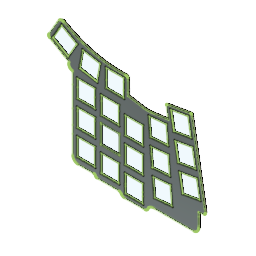
Klein-switchplate-MX-v2 (Autodesk Fusion 360 design; units mm, degrees)
Autodesk Fusion 360 part; units mm, degrees
note: some values were not read from the file. Set by a fixed rule: which sketch regions a step uses.
sketch "Sketch1" plane through (0, 0, 0) normal (0, 1, 0) x (1, 0, 0)
  line L0 (58.9921, 32.8367) -> (59.0035, 32.7548)
  line L1 (59.0035, 32.7548) -> (59.0201, 32.6338)
  line L2 (59.0201, 32.6338) -> (59.0381, 32.4299)
  line L3 (59.0381, 32.4299) -> (59.0461, 32.226)
  line L4 (59.0461, 32.226) -> (59.0441, 32.0221)
  line L5 (59.0441, 32.0221) -> (59.0321, 31.8171)
  line L6 (59.0321, 31.8171) -> (59.0321, 30.7985)
  line L7 (59.0321, 30.7985) -> (59.0321, 24.5661)
  line L8 (59.0321, 24.5661) -> (59.0321, 21.4739)
  line L9 (59.0321, 21.4739) -> (59.0321, 21.4713)
  line L10 (59.0321, 21.4713) -> (63.4304, 20.5717)
  line L11 (63.4304, 20.5717) -> (63.484, 20.5607)
  line L12 (63.484, 20.5607) -> (63.5246, 20.5516)
  line L13 (63.5246, 20.5516) -> (63.6297, 20.5186)
  line L14 (63.6297, 20.5186) -> (63.6613, 20.5077)
  line L15 (63.6613, 20.5077) -> (63.7388, 20.4717)
  line L16 (63.7388, 20.4717) -> (63.7582, 20.4627)
  line L17 (63.7582, 20.4627) -> (63.8502, 20.4087)
  line L18 (63.8502, 20.4087) -> (63.9371, 20.3458)
  line L19 (63.9371, 20.3458) -> (63.9921, 20.297)
  line L20 (63.9921, 20.297) -> (64.0199, 20.272)
  line L21 (64.0199, 20.272) -> (64.0577, 20.2321)
  line L22 (64.0577, 20.2321) -> (64.088, 20.1975)
  line L23 (64.088, 20.1975) -> (64.1341, 20.1404)
  line L24 (64.1341, 20.1404) -> (64.1528, 20.1129)
  line L25 (64.1528, 20.1129) -> (64.2105, 20.0188)
  line L26 (64.2105, 20.0188) -> (64.2396, 19.9588)
  line L27 (64.2396, 19.9588) -> (64.263, 19.9093)
  line L28 (64.263, 19.9093) -> (64.2884, 19.8399)
  line L29 (64.2884, 19.8399) -> (64.3024, 19.7918)
  line L30 (64.3024, 19.7918) -> (64.3258, 19.6942)
  line L31 (64.3258, 19.6942) -> (64.3308, 19.6611)
  line L32 (64.3308, 19.6611) -> (64.3404, 19.5786)
  line L33 (64.3404, 19.5786) -> (64.3423, 19.5287)
  line L34 (64.3423, 19.5287) -> (64.3409, 19.4276)
  line L35 (64.3409, 19.4276) -> (64.3369, 19.3861)
  line L36 (64.3369, 19.3861) -> (64.33, 19.3222)
  line L37 (64.33, 19.3222) -> (63.8116, 16.3774)
  line L38 (63.8116, 16.3774) -> (60.9284, 0)
  line L39 (60.9284, 0) -> (58.0453, -16.3774)
  line L40 (58.0453, -16.3774) -> (57.1727, -21.3338)
  line L41 (57.1727, -21.3338) -> (55.1621, -32.7548)
  line L42 (55.1621, -32.7548) -> (53.7066, -41.0228)
  line L43 (53.7066, -41.0228) -> (53.3844, -42.8527)
  line L44 (53.3844, -42.8527) -> (53.3634, -42.9266)
  line L45 (53.3634, -42.9266) -> (53.3314, -43.0046)
  line L46 (53.3314, -43.0046) -> (53.3208, -43.0234)
  line L47 (53.3208, -43.0234) -> (53.2878, -43.0776)
  line L48 (53.2878, -43.0776) -> (53.275, -43.0951)
  line L49 (53.275, -43.0951) -> (53.2462, -43.1322)
  line L50 (53.2462, -43.1322) -> (53.228, -43.1516)
  line L51 (53.228, -43.1516) -> (53.1702, -43.2062)
  line L52 (53.1702, -43.2062) -> (53.1662, -43.21)
  line L53 (53.1662, -43.21) -> (53.1318, -43.2341)
  line L54 (53.1318, -43.2341) -> (53.0976, -43.2589)
  line L55 (53.0976, -43.2589) -> (53.0931, -43.2622)
  line L56 (53.0931, -43.2622) -> (53.0223, -43.2972)
  line L57 (53.0223, -43.2972) -> (53.0051, -43.306)
  line L58 (53.0051, -43.306) -> (52.978, -43.3154)
  line L59 (52.978, -43.3154) -> (52.9326, -43.3305)
  line L60 (52.9326, -43.3305) -> (52.8646, -43.3455)
  line L61 (52.8646, -43.3455) -> (52.8384, -43.3477)
  line L62 (52.8384, -43.3477) -> (52.749, -43.3525)
  line L63 (52.749, -43.3525) -> (52.7347, -43.3525)
  line L64 (52.7347, -43.3525) -> (49.1321, -42.728)
  line L65 (49.1321, -42.728) -> (36.5731, -40.551)
  line L66 (36.5731, -40.551) -> (33.9933, -40.1038)
  line L67 (33.9933, -40.1038) -> (33.9483, -40.0888)
  line L68 (33.9483, -40.0888) -> (33.8709, -40.0528)
  line L69 (33.8709, -40.0528) -> (33.8623, -40.0488)
  line L70 (33.8623, -40.0488) -> (33.8273, -40.0261)
  line L71 (33.8273, -40.0261) -> (33.7881, -39.9931)
  line L72 (33.7881, -39.9931) -> (33.759, -39.9722)
  line L73 (33.759, -39.9722) -> (33.7375, -39.9488)
  line L74 (33.7375, -39.9488) -> (33.7004, -39.9069)
  line L75 (33.7004, -39.9069) -> (33.6654, -39.8569)
  line L76 (33.6654, -39.8569) -> (33.6284, -39.7849)
  line L77 (33.6284, -39.7849) -> (33.6014, -39.7089)
  line L78 (33.6014, -39.7089) -> (33.589, -39.6354)
  line L79 (33.589, -39.6354) -> (33.5834, -39.5998)
  line L80 (33.5834, -39.5998) -> (33.5903, -39.4981)
  line L81 (33.5903, -39.4981) -> (33.5906, -39.4728)
  line L82 (33.5906, -39.4728) -> (33.5931, -39.4558)
  line L83 (33.5931, -39.4558) -> (33.5934, -39.454)
  line L84 (33.5934, -39.454) -> (34.7453, -32.7548)
  line L85 (34.7453, -32.7548) -> (35.1918, -30.1578)
  line L86 (35.1918, -30.1578) -> (32.7548, -29.8255)
  line L87 (32.7548, -29.8255) -> (23.4475, -28.5565)
  line L88 (23.4475, -28.5565) -> (22.1161, -28.3575)
  line L89 (22.1161, -28.3575) -> (21.6487, -28.3112)
  line L90 (21.6487, -28.3112) -> (20.7756, -28.2246)
  line L91 (20.7756, -28.2246) -> (19.4311, -28.1586)
  line L92 (19.4311, -28.1586) -> (18.0847, -28.1576)
  line L93 (18.0847, -28.1576) -> (16.7402, -28.2246)
  line L94 (16.7402, -28.2246) -> (15.4008, -28.3565)
  line L95 (15.4008, -28.3565) -> (2.9558, -30.4057)
  line L96 (2.9558, -30.4057) -> (2.9358, -32.7548)
  line L97 (2.9358, -32.7548) -> (2.866, -40.9434)
  line L98 (2.866, -40.9434) -> (2.8498, -42.8427)
  line L99 (2.8498, -42.8427) -> (2.8019, -42.9236)
  line L100 (2.8019, -42.9236) -> (2.7566, -42.9906)
  line L101 (2.7566, -42.9906) -> (2.7229, -43.0406)
  line L102 (2.7229, -43.0406) -> (2.6359, -43.1526)
  line L103 (2.6359, -43.1526) -> (2.5926, -43.2007)
  line L104 (2.5926, -43.2007) -> (2.5523, -43.2438)
  line L105 (2.5523, -43.2438) -> (2.507, -43.2905)
  line L106 (2.507, -43.2905) -> (2.402, -43.3845)
  line L107 (2.402, -43.3845) -> (2.2901, -43.4714)
  line L108 (2.2901, -43.4714) -> (2.1721, -43.5494)
  line L109 (2.1721, -43.5494) -> (2.0482, -43.6184)
  line L110 (2.0482, -43.6184) -> (2.0472, -43.6188)
  line L111 (2.0472, -43.6188) -> (2.0216, -43.6312)
  line L112 (2.0216, -43.6312) -> (1.9034, -43.6848)
  line L113 (1.9034, -43.6848) -> (1.8488, -43.7063)
  line L114 (1.8488, -43.7063) -> (1.7883, -43.7283)
  line L115 (1.7883, -43.7283) -> (1.6523, -43.7683)
  line L116 (1.6523, -43.7683) -> (1.5144, -43.7993)
  line L117 (1.5144, -43.7993) -> (1.3734, -43.8183)
  line L118 (1.3734, -43.8183) -> (1.2325, -43.8283)
  line L119 (1.2325, -43.8283) -> (1.0916, -43.8263)
  line L120 (1.0916, -43.8263) -> (0.9506, -43.8153)
  line L121 (0.9506, -43.8153) -> (0.8567, -43.8013)
  line L122 (0.8567, -43.8013) -> (0.7395, -43.7988)
  line L123 (0.7395, -43.7988) -> (0, -43.7832)
  line L124 (0, -43.7832) -> (-3.3556, -43.7123)
  line L125 (-3.3556, -43.7123) -> (-7.5679, -43.8223)
  line L126 (-7.5679, -43.8223) -> (-11.7702, -44.1302)
  line L127 (-11.7702, -44.1302) -> (-15.9535, -44.637)
  line L128 (-15.9535, -44.637) -> (-20.1079, -45.3407)
  line L129 (-20.1079, -45.3407) -> (-24.2242, -46.2403)
  line L130 (-24.2242, -46.2403) -> (-28.2936, -47.3329)
  line L131 (-28.2936, -47.3329) -> (-32.3069, -48.6163)
  line L132 (-32.3069, -48.6163) -> (-32.7548, -48.7832)
  line L133 (-32.7548, -48.7832) -> (-33.691, -49.1321)
  line L134 (-33.691, -49.1321) -> (-36.2553, -50.0877)
  line L135 (-36.2553, -50.0877) -> (-40.1298, -51.7441)
  line L136 (-40.1298, -51.7441) -> (-43.9222, -53.5823)
  line L137 (-43.9222, -53.5823) -> (-47.6227, -55.5975)
  line L138 (-47.6227, -55.5975) -> (-47.7467, -55.6825)
  line L139 (-47.7467, -55.6825) -> (-47.9406, -55.7984)
  line L140 (-47.9406, -55.7984) -> (-48.1415, -55.9014)
  line L141 (-48.1415, -55.9014) -> (-48.2893, -55.9605)
  line L142 (-48.2893, -55.9605) -> (-48.334, -55.9784)
  line L143 (-48.334, -55.9784) -> (-48.3774, -55.9968)
  line L144 (-48.3774, -55.9968) -> (-48.3976, -56.0038)
  line L145 (-48.3976, -56.0038) -> (-48.4664, -56.0277)
  line L146 (-48.4664, -56.0277) -> (-48.5654, -56.0593)
  line L147 (-48.5654, -56.0593) -> (-48.7843, -56.1133)
  line L148 (-48.7843, -56.1133) -> (-49.0072, -56.1533)
  line L149 (-49.0072, -56.1533) -> (-49.1321, -56.1641)
  line L150 (-49.1321, -56.1641) -> (-49.3071, -56.1793)
  line L151 (-49.3071, -56.1793) -> (-49.533, -56.1783)
  line L152 (-49.533, -56.1783) -> (-49.7579, -56.1633)
  line L153 (-49.7579, -56.1633) -> (-49.9818, -56.1293)
  line L154 (-49.9818, -56.1293) -> (-50.2027, -56.0813)
  line L155 (-50.2027, -56.0813) -> (-50.3476, -56.0393)
  line L156 (-50.3476, -56.0393) -> (-50.5596, -55.9624)
  line L157 (-50.5596, -55.9624) -> (-50.7665, -55.8714)
  line L158 (-50.7665, -55.8714) -> (-50.8083, -55.8499)
  line L159 (-50.8083, -55.8499) -> (-50.9898, -55.7502)
  line L160 (-50.9898, -55.7502) -> (-51.0304, -55.7265)
  line L161 (-51.0304, -55.7265) -> (-51.2183, -55.6005)
  line L162 (-51.2183, -55.6005) -> (-51.3972, -55.4626)
  line L163 (-51.3972, -55.4626) -> (-51.6181, -55.2577)
  line L164 (-51.6181, -55.2577) -> (-51.7201, -55.1467)
  line L165 (-51.7201, -55.1467) -> (-52.8694, -53.2265)
  line L166 (-52.8694, -53.2265) -> (-53.2265, -52.6299)
  line L167 (-53.2265, -52.6299) -> (-55.32, -49.1321)
  line L168 (-55.32, -49.1321) -> (-59.6169, -41.953)
  line L169 (-59.6169, -41.953) -> (-59.6669, -41.8851)
  line L170 (-59.6669, -41.8851) -> (-59.7348, -41.7801)
  line L171 (-59.7348, -41.7801) -> (-59.8138, -41.6322)
  line L172 (-59.8138, -41.6322) -> (-59.8638, -41.5162)
  line L173 (-59.8638, -41.5162) -> (-59.8725, -41.4915)
  line L174 (-59.8725, -41.4915) -> (-59.9152, -41.3541)
  line L175 (-59.9152, -41.3541) -> (-59.9258, -41.3163)
  line L176 (-59.9258, -41.3163) -> (-59.9518, -41.1933)
  line L177 (-59.9518, -41.1933) -> (-59.9678, -41.0694)
  line L178 (-59.9678, -41.0694) -> (-59.9758, -40.9434)
  line L179 (-59.9758, -40.9434) -> (-59.9728, -40.8185)
  line L180 (-59.9728, -40.8185) -> (-59.9696, -40.7791)
  line L181 (-59.9696, -40.7791) -> (-59.9579, -40.6644)
  line L182 (-59.9579, -40.6644) -> (-59.9539, -40.6388)
  line L183 (-59.9539, -40.6388) -> (-59.9312, -40.5261)
  line L184 (-59.9312, -40.5261) -> (-59.9228, -40.4876)
  line L185 (-59.9228, -40.4876) -> (-59.8868, -40.3667)
  line L186 (-59.8868, -40.3667) -> (-59.8675, -40.3124)
  line L187 (-59.8675, -40.3124) -> (-59.8485, -40.2637)
  line L188 (-59.8485, -40.2637) -> (-59.8134, -40.1846)
  line L189 (-59.8134, -40.1846) -> (-59.7959, -40.1496)
  line L190 (-59.7959, -40.1496) -> (-59.7561, -40.0734)
  line L191 (-59.7561, -40.0734) -> (-59.7361, -40.0393)
  line L192 (-59.7361, -40.0393) -> (-59.6564, -39.9197)
  line L193 (-59.6564, -39.9197) -> (-59.6339, -39.8879)
  line L194 (-59.6339, -39.8879) -> (-59.5549, -39.7899)
  line L195 (-59.5549, -39.7899) -> (-59.468, -39.6989)
  line L196 (-59.468, -39.6989) -> (-59.376, -39.614)
  line L197 (-59.376, -39.614) -> (-59.3451, -39.5896)
  line L198 (-59.3451, -39.5896) -> (-59.2537, -39.5195)
  line L199 (-59.2537, -39.5195) -> (-59.2212, -39.4977)
  line L200 (-59.2212, -39.4977) -> (-59.1229, -39.4372)
  line L201 (-59.1229, -39.4372) -> (-59.1001, -39.4241)
  line L202 (-59.1001, -39.4241) -> (-57.3208, -38.4036)
  line L203 (-57.3208, -38.4036) -> (-49.1321, -33.7073)
  line L204 (-49.1321, -33.7073) -> (-47.4712, -32.7548)
  line L205 (-47.4712, -32.7548) -> (-43.5914, -30.5297)
  line L206 (-43.5914, -30.5297) -> (-43.6993, -30.3187)
  line L207 (-43.6993, -30.3187) -> (-43.729, -30.2506)
  line L208 (-43.729, -30.2506) -> (-43.8128, -30.0493)
  line L209 (-43.8128, -30.0493) -> (-43.8366, -29.9787)
  line L210 (-43.8366, -29.9787) -> (-43.8861, -29.8227)
  line L211 (-43.8861, -29.8227) -> (-43.9051, -29.7508)
  line L212 (-43.9051, -29.7508) -> (-43.9312, -29.645)
  line L213 (-43.9312, -29.645) -> (-43.9732, -29.4111)
  line L214 (-43.9732, -29.4111) -> (-43.9813, -29.3374)
  line L215 (-43.9813, -29.3374) -> (-44.002, -29.1209)
  line L216 (-44.002, -29.1209) -> (-44.0041, -29.0712)
  line L217 (-44.0041, -29.0712) -> (-44.0028, -28.8534)
  line L218 (-44.0028, -28.8534) -> (-44.0012, -28.7794)
  line L219 (-44.0012, -28.7794) -> (-43.9943, -28.7053)
  line L220 (-43.9943, -28.7053) -> (-43.9895, -28.6604)
  line L221 (-43.9895, -28.6604) -> (-43.971, -28.4882)
  line L222 (-43.971, -28.4882) -> (-43.9635, -28.4391)
  line L223 (-43.9635, -28.4391) -> (-43.9188, -28.2261)
  line L224 (-43.9188, -28.2261) -> (-43.9022, -28.1536)
  line L225 (-43.9022, -28.1536) -> (-43.8555, -27.9969)
  line L226 (-43.8555, -27.9969) -> (-43.8287, -27.9118)
  line L227 (-43.8287, -27.9118) -> (-43.8258, -27.9026)
  line L228 (-43.8258, -27.9026) -> (-43.7977, -27.8339)
  line L229 (-43.7977, -27.8339) -> (-43.7173, -27.6318)
  line L230 (-43.7173, -27.6318) -> (-43.6163, -27.438)
  line L231 (-43.6163, -27.438) -> (-43.5823, -27.3718)
  line L232 (-43.5823, -27.3718) -> (-43.5793, -27.367)
  line L233 (-43.5793, -27.367) -> (-43.5301, -27.2875)
  line L234 (-43.5301, -27.2875) -> (-43.4105, -27.1054)
  line L235 (-43.4105, -27.1054) -> (-43.3343, -27.0079)
  line L236 (-43.3343, -27.0079) -> (-43.2683, -26.9213)
  line L237 (-43.2683, -26.9213) -> (-43.2529, -26.9039)
  line L238 (-43.2529, -26.9039) -> (-43.1604, -26.799)
  line L239 (-43.1604, -26.799) -> (-43.1086, -26.7459)
  line L240 (-43.1086, -26.7459) -> (-43.0247, -26.6625)
  line L241 (-43.0247, -26.6625) -> (-42.9924, -26.6304)
  line L242 (-42.9924, -26.6304) -> (-42.9726, -26.6132)
  line L243 (-42.9726, -26.6132) -> (-42.91, -26.5589)
  line L244 (-42.91, -26.5589) -> (-42.7801, -26.46)
  line L245 (-42.7801, -26.46) -> (-42.6657, -26.3653)
  line L246 (-42.6657, -26.3653) -> (-42.529, -26.2753)
  line L247 (-42.529, -26.2753) -> (-42.511, -26.2639)
  line L248 (-42.511, -26.2639) -> (-42.4453, -26.2222)
  line L249 (-42.4453, -26.2222) -> (-42.3511, -26.1679)
  line L250 (-42.3511, -26.1679) -> (-42.1539, -26.0751)
  line L251 (-42.1539, -26.0751) -> (-42.0883, -26.0405)
  line L252 (-42.0883, -26.0405) -> (-42.043, -26.0205)
  line L253 (-42.043, -26.0205) -> (-41.8201, -25.9385)
  line L254 (-41.8201, -25.9385) -> (-41.6119, -25.8776)
  line L255 (-41.6119, -25.8776) -> (-41.5912, -25.8715)
  line L256 (-41.5912, -25.8715) -> (-41.3775, -25.8303)
  line L257 (-41.3775, -25.8303) -> (-41.3047, -25.8156)
  line L258 (-41.3047, -25.8156) -> (-41.2063, -25.8041)
  line L259 (-41.2063, -25.8041) -> (-41.0434, -25.7876)
  line L260 (-41.0434, -25.7876) -> (-40.9434, -25.7842)
  line L261 (-40.9434, -25.7842) -> (-40.8065, -25.7796)
  line L262 (-40.8065, -25.7796) -> (-40.8065, -24.5661)
  line L263 (-40.8065, -24.5661) -> (-40.8068, -16.3774)
  line L264 (-40.8068, -16.3774) -> (-40.8074, 0)
  line L265 (-40.8074, 0) -> (-40.8078, 11.4254)
  line L266 (-40.8078, 11.4254) -> (-40.808, 17.5229)
  line L267 (-40.808, 17.5229) -> (-40.8085, 31.5173)
  line L268 (-40.8085, 31.5173) -> (-40.8085, 32.167)
  line L269 (-40.8085, 32.167) -> (-40.8055, 32.3709)
  line L270 (-40.8055, 32.3709) -> (-40.7925, 32.5738)
  line L271 (-40.7925, 32.5738) -> (-40.772, 32.7548)
  line L272 (-40.772, 32.7548) -> (-40.7695, 32.7767)
  line L273 (-40.7695, 32.7767) -> (-40.7355, 32.9777)
  line L274 (-40.7355, 32.9777) -> (-40.6925, 33.1766)
  line L275 (-40.6925, 33.1766) -> (-40.6406, 33.3735)
  line L276 (-40.6406, 33.3735) -> (-40.5776, 33.5674)
  line L277 (-40.5776, 33.5674) -> (-40.5056, 33.7574)
  line L278 (-40.5056, 33.7574) -> (-40.4237, 33.9443)
  line L279 (-40.4237, 33.9443) -> (-40.3337, 34.1262)
  line L280 (-40.3337, 34.1262) -> (-40.2337, 34.3041)
  line L281 (-40.2337, 34.3041) -> (-40.1258, 34.4771)
  line L282 (-40.1258, 34.4771) -> (-40.0088, 34.644)
  line L283 (-40.0088, 34.644) -> (-39.8872, 34.8019)
  line L284 (-39.8872, 34.8019) -> (-39.8849, 34.8049)
  line L285 (-39.8849, 34.8049) -> (-39.7519, 34.9599)
  line L286 (-39.7519, 34.9599) -> (-39.612, 35.1068)
  line L287 (-39.612, 35.1068) -> (-39.465, 35.2477)
  line L288 (-39.465, 35.2477) -> (-39.3101, 35.3807)
  line L289 (-39.3101, 35.3807) -> (-39.1502, 35.5066)
  line L290 (-39.1502, 35.5066) -> (-38.9832, 35.6236)
  line L291 (-38.9832, 35.6236) -> (-38.8963, 35.6787)
  line L292 (-38.8963, 35.6787) -> (-38.8113, 35.7326)
  line L293 (-38.8113, 35.7326) -> (-38.6344, 35.8325)
  line L294 (-38.6344, 35.8325) -> (-38.4525, 35.9245)
  line L295 (-38.4525, 35.9245) -> (-38.2655, 36.0064)
  line L296 (-38.2655, 36.0064) -> (-38.0756, 36.0794)
  line L297 (-38.0756, 36.0794) -> (-37.8827, 36.1424)
  line L298 (-37.8827, 36.1424) -> (-37.6858, 36.1964)
  line L299 (-37.6858, 36.1964) -> (-37.4868, 36.2403)
  line L300 (-37.4868, 36.2403) -> (-37.2859, 36.2743)
  line L301 (-37.2859, 36.2743) -> (-37.084, 36.2983)
  line L302 (-37.084, 36.2983) -> (-36.8811, 36.3123)
  line L303 (-36.8811, 36.3123) -> (-36.8491, 36.3128)
  line L304 (-36.8491, 36.3128) -> (-36.6772, 36.3153)
  line L305 (-36.6772, 36.3153) -> (-32.7548, 36.3153)
  line L306 (-32.7548, 36.3153) -> (-24.5661, 36.3153)
  line L307 (-24.5661, 36.3153) -> (-24.2322, 36.3153)
  line L308 (-24.2322, 36.3153) -> (-24.1649, 36.3126)
  line L309 (-24.1649, 36.3126) -> (-24.1239, 36.3113)
  line L310 (-24.1239, 36.3113) -> (-24.0559, 36.3134)
  line L311 (-24.0559, 36.3134) -> (-24.039, 36.3153)
  line L312 (-24.039, 36.3153) -> (-23.9744, 36.3228)
  line L313 (-23.9744, 36.3228) -> (-23.8404, 36.3413)
  line L314 (-23.8404, 36.3413) -> (-23.8104, 36.3491)
  line L315 (-23.8104, 36.3491) -> (-23.6805, 36.3883)
  line L316 (-23.6805, 36.3883) -> (-23.6561, 36.3967)
  line L317 (-23.6561, 36.3967) -> (-23.6514, 36.3983)
  line L318 (-23.6514, 36.3983) -> (-23.5905, 36.4233)
  line L319 (-23.5905, 36.4233) -> (-23.4702, 36.4865)
  line L320 (-23.4702, 36.4865) -> (-23.4424, 36.4999)
  line L321 (-23.4424, 36.4999) -> (-23.4071, 36.5209)
  line L322 (-23.4071, 36.5209) -> (-23.2985, 36.6013)
  line L323 (-23.2985, 36.6013) -> (-23.2576, 36.6322)
  line L324 (-23.2576, 36.6322) -> (-23.1177, 36.7721)
  line L325 (-23.1177, 36.7721) -> (-23.0757, 36.8231)
  line L326 (-23.0757, 36.8231) -> (-23.0584, 36.8491)
  line L327 (-23.0584, 36.8491) -> (-22.9667, 36.987)
  line L328 (-22.9667, 36.987) -> (-22.9454, 37.0269)
  line L329 (-22.9454, 37.0269) -> (-22.9314, 37.0544)
  line L330 (-22.9314, 37.0544) -> (-22.9151, 37.0911)
  line L331 (-22.9151, 37.0911) -> (-22.9039, 37.1162)
  line L332 (-22.9039, 37.1162) -> (-22.8917, 37.1444)
  line L333 (-22.8917, 37.1444) -> (-22.8573, 37.2358)
  line L334 (-22.8573, 37.2358) -> (-22.832, 37.2992)
  line L335 (-22.832, 37.2992) -> (-22.8018, 37.3679)
  line L336 (-22.8018, 37.3679) -> (-22.7318, 37.4948)
  line L337 (-22.7318, 37.4948) -> (-22.6718, 37.5848)
  line L338 (-22.6718, 37.5848) -> (-22.5819, 37.6988)
  line L339 (-22.5819, 37.6988) -> (-22.5189, 37.7659)
  line L340 (-22.5189, 37.7659) -> (-22.5069, 37.7787)
  line L341 (-22.5069, 37.7787) -> (-22.3989, 37.8757)
  line L342 (-22.3989, 37.8757) -> (-22.3718, 37.896)
  line L343 (-22.3718, 37.896) -> (-22.2494, 37.9819)
  line L344 (-22.2494, 37.9819) -> (-22.221, 38.0006)
  line L345 (-22.221, 38.0006) -> (-22.087, 38.068)
  line L346 (-22.087, 38.068) -> (-22.0158, 38.1027)
  line L347 (-22.0158, 38.1027) -> (-21.9697, 38.1205)
  line L348 (-21.9697, 38.1205) -> (-21.8983, 38.1432)
  line L349 (-21.8983, 38.1432) -> (-21.8442, 38.1607)
  line L350 (-21.8442, 38.1607) -> (-21.8405, 38.1615)
  line L351 (-21.8405, 38.1615) -> (-21.7245, 38.1877)
  line L352 (-21.7245, 38.1877) -> (-21.691, 38.193)
  line L353 (-21.691, 38.193) -> (-21.6175, 38.204)
  line L354 (-21.6175, 38.204) -> (-21.5835, 38.2074)
  line L355 (-21.5835, 38.2074) -> (-21.5333, 38.2116)
  line L356 (-21.5333, 38.2116) -> (-20.4717, 38.2117)
  line L357 (-20.4717, 38.2117) -> (-16.3774, 38.2124)
  line L358 (-16.3774, 38.2124) -> (-8.1887, 38.2139)
  line L359 (-8.1887, 38.2139) -> (-4.2413, 38.2145)
  line L360 (-4.2413, 38.2145) -> (-4.0943, 38.2406)
  line L361 (-4.0943, 38.2406) -> (-4.0384, 38.2505)
  line L362 (-4.0384, 38.2505) -> (-3.8394, 38.2995)
  line L363 (-3.8394, 38.2995) -> (-3.7494, 38.3277)
  line L364 (-3.7494, 38.3277) -> (-3.6685, 38.3555)
  line L365 (-3.6685, 38.3555) -> (-3.494, 38.4256)
  line L366 (-3.494, 38.4256) -> (-3.4546, 38.4425)
  line L367 (-3.4546, 38.4425) -> (-3.2717, 38.5344)
  line L368 (-3.2717, 38.5344) -> (-3.0947, 38.6394)
  line L369 (-3.0947, 38.6394) -> (-2.9818, 38.7173)
  line L370 (-2.9818, 38.7173) -> (-2.8209, 38.8443)
  line L371 (-2.8209, 38.8443) -> (-2.7647, 38.8963)
  line L372 (-2.7647, 38.8963) -> (-2.6199, 39.0302)
  line L373 (-2.6199, 39.0302) -> (-2.482, 39.1822)
  line L374 (-2.482, 39.1822) -> (-2.4551, 39.2156)
  line L375 (-2.4551, 39.2156) -> (-2.407, 39.2859)
  line L376 (-2.407, 39.2859) -> (-2.3359, 39.3793)
  line L377 (-2.3359, 39.3793) -> (-2.2929, 39.4357)
  line L378 (-2.2929, 39.4357) -> (-2.2421, 39.514)
  line L379 (-2.2421, 39.514) -> (-2.2218, 39.5518)
  line L380 (-2.2218, 39.5518) -> (-2.208, 39.5767)
  line L381 (-2.208, 39.5767) -> (-2.1531, 39.6755)
  line L382 (-2.1531, 39.6755) -> (-2.1193, 39.7302)
  line L383 (-2.1193, 39.7302) -> (-2.0437, 39.8491)
  line L384 (-2.0437, 39.8491) -> (-2.0066, 39.9012)
  line L385 (-2.0066, 39.9012) -> (-1.9502, 39.9768)
  line L386 (-1.9502, 39.9768) -> (-1.8697, 40.0709)
  line L387 (-1.8697, 40.0709) -> (-1.7723, 40.1848)
  line L388 (-1.7723, 40.1848) -> (-1.6243, 40.3277)
  line L389 (-1.6243, 40.3277) -> (-1.4684, 40.4606)
  line L390 (-1.4684, 40.4606) -> (-1.3015, 40.5806)
  line L391 (-1.3015, 40.5806) -> (-1.1275, 40.6886)
  line L392 (-1.1275, 40.6886) -> (-0.8826, 40.8125)
  line L393 (-0.8826, 40.8125) -> (-0.6917, 40.8875)
  line L394 (-0.6917, 40.8875) -> (-0.5185, 40.9434)
  line L395 (-0.5185, 40.9434) -> (-0.4968, 40.9504)
  line L396 (-0.4968, 40.9504) -> (-0.3639, 40.9834)
  line L397 (-0.3639, 40.9834) -> (0, 40.9813)
  line L398 (0, 40.9813) -> (0.8167, 40.9764)
  line L399 (0.8167, 40.9764) -> (14.811, 40.8933)
  line L400 (14.811, 40.8933) -> (16.3774, 40.884)
  line L401 (16.3774, 40.884) -> (16.4713, 40.8835)
  line L402 (16.4713, 40.8835) -> (16.7072, 40.8755)
  line L403 (16.7072, 40.8755) -> (16.8822, 40.8545)
  line L404 (16.8822, 40.8545) -> (17.0561, 40.8215)
  line L405 (17.0561, 40.8215) -> (17.092, 40.8121)
  line L406 (17.092, 40.8121) -> (17.2487, 40.7681)
  line L407 (17.2487, 40.7681) -> (17.3012, 40.751)
  line L408 (17.3012, 40.751) -> (17.3524, 40.7307)
  line L409 (17.3524, 40.7307) -> (17.5029, 40.6716)
  line L410 (17.5029, 40.6716) -> (17.5084, 40.6688)
  line L411 (17.5084, 40.6688) -> (17.6619, 40.5926)
  line L412 (17.6619, 40.5926) -> (17.8148, 40.5036)
  line L413 (17.8148, 40.5036) -> (18.0077, 40.3677)
  line L414 (18.0077, 40.3677) -> (18.1427, 40.2527)
  line L415 (18.1427, 40.2527) -> (18.2696, 40.1298)
  line L416 (18.2696, 40.1298) -> (18.3866, 39.9968)
  line L417 (18.3866, 39.9968) -> (18.4245, 39.9476)
  line L418 (18.4245, 39.9476) -> (18.4945, 39.8569)
  line L419 (18.4945, 39.8569) -> (18.5905, 39.7079)
  line L420 (18.5905, 39.7079) -> (18.6336, 39.6264)
  line L421 (18.6336, 39.6264) -> (18.6934, 39.5206)
  line L422 (18.6934, 39.5206) -> (18.7284, 39.4471)
  line L423 (18.7284, 39.4471) -> (18.7944, 39.2831)
  line L424 (18.7944, 39.2831) -> (18.8288, 39.1822)
  line L425 (18.8288, 39.1822) -> (18.8666, 39.0661)
  line L426 (18.8666, 39.0661) -> (18.9315, 38.8963)
  line L427 (18.9315, 38.8963) -> (18.947, 38.8558)
  line L428 (18.947, 38.8558) -> (18.9773, 38.7852)
  line L429 (18.9773, 38.7852) -> (19.0515, 38.6333)
  line L430 (19.0515, 38.6333) -> (19.0862, 38.5649)
  line L431 (19.0862, 38.5649) -> (19.1693, 38.4178)
  line L432 (19.1693, 38.4178) -> (19.2234, 38.3307)
  line L433 (19.2234, 38.3307) -> (19.2548, 38.2828)
  line L434 (19.2548, 38.2828) -> (19.2852, 38.2365)
  line L435 (19.2852, 38.2365) -> (19.3471, 38.155)
  line L436 (19.3471, 38.155) -> (19.413, 38.0636)
  line L437 (19.413, 38.0636) -> (19.5573, 37.8911)
  line L438 (19.5573, 37.8911) -> (19.5911, 37.8527)
  line L439 (19.5911, 37.8527) -> (19.6639, 37.7805)
  line L440 (19.6639, 37.7805) -> (19.7422, 37.6994)
  line L441 (19.7422, 37.6994) -> (19.7803, 37.6651)
  line L442 (19.7803, 37.6651) -> (19.9099, 37.5483)
  line L443 (19.9099, 37.5483) -> (19.9489, 37.5148)
  line L444 (19.9489, 37.5148) -> (20.1648, 37.3549)
  line L445 (20.1648, 37.3549) -> (20.3888, 37.206)
  line L446 (20.3888, 37.206) -> (20.4717, 37.1555)
  line L447 (20.4717, 37.1555) -> (20.6187, 37.066)
  line L448 (20.6187, 37.066) -> (20.8556, 36.9381)
  line L449 (20.8556, 36.9381) -> (21.0412, 36.8491)
  line L450 (21.0412, 36.8491) -> (21.0975, 36.8221)
  line L451 (21.0975, 36.8221) -> (21.3454, 36.7172)
  line L452 (21.3454, 36.7172) -> (21.5983, 36.6232)
  line L453 (21.5983, 36.6232) -> (21.8542, 36.5422)
  line L454 (21.8542, 36.5422) -> (22.1141, 36.4733)
  line L455 (22.1141, 36.4733) -> (22.377, 36.4163)
  line L456 (22.377, 36.4163) -> (22.6428, 36.3723)
  line L457 (22.6428, 36.3723) -> (22.9097, 36.3413)
  line L458 (22.9097, 36.3413) -> (23.1786, 36.3223)
  line L459 (23.1786, 36.3223) -> (23.4475, 36.3153)
  line L460 (23.4475, 36.3153) -> (24.5661, 36.3153)
  line L461 (24.5661, 36.3153) -> (32.7548, 36.3153)
  line L462 (32.7548, 36.3153) -> (49.1321, 36.3153)
  line L463 (49.1321, 36.3153) -> (55.2297, 36.3153)
  line L464 (55.2297, 36.3153) -> (55.4326, 36.2933)
  line L465 (55.4326, 36.2933) -> (55.6345, 36.2613)
  line L466 (55.6345, 36.2613) -> (55.8344, 36.2204)
  line L467 (55.8344, 36.2204) -> (56.0323, 36.1684)
  line L468 (56.0323, 36.1684) -> (56.2273, 36.1074)
  line L469 (56.2273, 36.1074) -> (56.4192, 36.0364)
  line L470 (56.4192, 36.0364) -> (56.6071, 35.9565)
  line L471 (56.6071, 35.9565) -> (56.791, 35.8665)
  line L472 (56.791, 35.8665) -> (56.971, 35.7685)
  line L473 (56.971, 35.7685) -> (57.1449, 35.6616)
  line L474 (57.1449, 35.6616) -> (57.3138, 35.5466)
  line L475 (57.3138, 35.5466) -> (57.3208, 35.5413)
  line L476 (57.3208, 35.5413) -> (57.4768, 35.4237)
  line L477 (57.4768, 35.4237) -> (57.6337, 35.2917)
  line L478 (57.6337, 35.2917) -> (57.7836, 35.1528)
  line L479 (57.7836, 35.1528) -> (57.9266, 35.0068)
  line L480 (57.9266, 35.0068) -> (58.0625, 34.8539)
  line L481 (58.0625, 34.8539) -> (58.1044, 34.8019)
  line L482 (58.1044, 34.8019) -> (58.1905, 34.695)
  line L483 (58.1905, 34.695) -> (58.3104, 34.53)
  line L484 (58.3104, 34.53) -> (58.4224, 34.3581)
  line L485 (58.4224, 34.3581) -> (58.5263, 34.1822)
  line L486 (58.5263, 34.1822) -> (58.6203, 34.0013)
  line L487 (58.6203, 34.0013) -> (58.7063, 33.8153)
  line L488 (58.7063, 33.8153) -> (58.7822, 33.6254)
  line L489 (58.7822, 33.6254) -> (58.8492, 33.4325)
  line L490 (58.8492, 33.4325) -> (58.9072, 33.2366)
  line L491 (58.9072, 33.2366) -> (58.9542, 33.0376)
  line L492 (58.9542, 33.0376) -> (58.9921, 32.8367)
  line L493 (43.9522, 1.2975) -> (51.3106, 0)
  line L494 (51.3106, 0) -> (57.7337, -1.1325)
  line L495 (57.7337, -1.1325) -> (57.9333, 0)
  line L496 (57.9333, 0) -> (60.1637, 12.6499)
  line L497 (60.1637, 12.6499) -> (46.3822, 15.0799)
  line L498 (46.3822, 15.0799) -> (43.9522, 1.2975)
  line L499 (0.8167, 31.084) -> (0.8167, 23.8204)
  line L500 (0.8167, 23.8204) -> (14.811, 23.8204)
  line L501 (14.811, 23.8204) -> (14.811, 29.8598)
  line L502 (14.811, 29.8598) -> (14.811, 32.7548)
  line L503 (14.811, 32.7548) -> (14.811, 37.8147)
  line L504 (14.811, 37.8147) -> (0.8167, 37.8147)
  line L505 (0.8167, 37.8147) -> (0.8167, 32.7548)
  line L506 (0.8167, 32.7548) -> (0.8167, 31.084)
  line L507 (-23.1726, -8.5665) -> (-32.7548, -8.5665)
  line L508 (-32.7548, -8.5665) -> (-37.167, -8.5665)
  line L509 (-37.167, -8.5665) -> (-37.167, -16.3774)
  line L510 (-37.167, -16.3774) -> (-37.167, -22.5609)
  line L511 (-37.167, -22.5609) -> (-32.7548, -22.5609)
  line L512 (-32.7548, -22.5609) -> (-23.1726, -22.5609)
  line L513 (-23.1726, -22.5609) -> (-23.1726, -16.3774)
  line L514 (-23.1726, -16.3774) -> (-23.1726, -8.5665)
  line L515 (37.9936, 27.8317) -> (32.7548, 28.29)
  line L516 (32.7548, 28.29) -> (24.0533, 29.0513)
  line L517 (24.0533, 29.0513) -> (22.8338, 15.1109)
  line L518 (22.8338, 15.1109) -> (32.7548, 14.243)
  line L519 (32.7548, 14.243) -> (36.7741, 13.8914)
  line L520 (36.7741, 13.8914) -> (36.9916, 16.3774)
  line L521 (36.9916, 16.3774) -> (37.9936, 27.8317)
  line L522 (32.7548, 8.2219) -> (22.3111, 9.1363)
  line L523 (22.3111, 9.1363) -> (22.311, 9.1363)
  line L524 (22.311, 9.1363) -> (21.8467, 3.8285)
  line L525 (21.8467, 3.8285) -> (21.5118, 0)
  line L526 (21.5118, 0) -> (21.0915, -4.8051)
  line L527 (21.0915, -4.8051) -> (32.7548, -5.8254)
  line L528 (32.7548, -5.8254) -> (35.0318, -6.0246)
  line L529 (35.0318, -6.0246) -> (35.5589, 0)
  line L530 (35.5589, 0) -> (36.2513, 7.9158)
  line L531 (36.2513, 7.9158) -> (32.7548, 8.2219)
  line L532 (14.811, 17.8228) -> (0.8167, 17.8228)
  line L533 (0.8167, 17.8228) -> (0.8167, 3.8285)
  line L534 (0.8167, 3.8285) -> (14.811, 3.8285)
  line L535 (14.811, 3.8285) -> (14.811, 17.8228)
  line L536 (56.6921, -7.0382) -> (42.9107, -4.6081)
  line L537 (42.9107, -4.6081) -> (41.4513, -12.885)
  line L538 (41.4513, -12.885) -> (40.8356, -16.3774)
  line L539 (40.8356, -16.3774) -> (40.4806, -18.3906)
  line L540 (40.4806, -18.3906) -> (54.262, -20.8206)
  line L541 (54.262, -20.8206) -> (55.0455, -16.3774)
  line L542 (55.0455, -16.3774) -> (56.6921, -7.0382)
  line L543 (32.7548, -12.1242) -> (20.8356, -11.0815)
  line L544 (20.8356, -11.0815) -> (20.3719, -16.3774)
  line L545 (20.3719, -16.3774) -> (19.6151, -25.0229)
  line L546 (19.6151, -25.0229) -> (32.7548, -26.1723)
  line L547 (32.7548, -26.1723) -> (33.5564, -26.2424)
  line L548 (33.5564, -26.2424) -> (34.4194, -16.3774)
  line L549 (34.4194, -16.3774) -> (34.7759, -12.301)
  line L550 (34.7759, -12.301) -> (34.485, -12.2756)
  line L551 (34.485, -12.2756) -> (32.7548, -12.1242)
  line L552 (53.2205, -26.7272) -> (39.4391, -24.2972)
  line L553 (39.4391, -24.2972) -> (39.0119, -26.7196)
  line L554 (39.0119, -26.7196) -> (38.3302, -30.5857)
  line L555 (38.3302, -30.5857) -> (37.9478, -32.7548)
  line L556 (37.9478, -32.7548) -> (37.009, -38.0786)
  line L557 (37.009, -38.0786) -> (49.1321, -40.2162)
  line L558 (49.1321, -40.2162) -> (50.7905, -40.5086)
  line L559 (50.7905, -40.5086) -> (52.1577, -32.7548)
  line L560 (52.1577, -32.7548) -> (53.2205, -26.7272)
  line L561 (0.8167, -16.1635) -> (14.811, -16.1635)
  line L562 (14.811, -16.1635) -> (14.811, -2.1691)
  line L563 (14.811, -2.1691) -> (0.8167, -2.1691)
  line L564 (0.8167, -2.1691) -> (0.8167, -16.1635)
  line L565 (-4.1813, 33.4165) -> (-8.1887, 33.4165)
  line L566 (-8.1887, 33.4165) -> (-16.3774, 33.4165)
  line L567 (-16.3774, 33.4165) -> (-18.1747, 33.4165)
  line L568 (-18.1747, 33.4165) -> (-18.1747, 32.7548)
  line L569 (-18.1747, 32.7548) -> (-18.1747, 19.4221)
  line L570 (-18.1747, 19.4221) -> (-4.1813, 19.4221)
  line L571 (-4.1813, 19.4221) -> (-4.1813, 32.7548)
  line L572 (-4.1813, 32.7548) -> (-4.1813, 33.4165)
  line L573 (-3.6275, 13.4246) -> (-3.6275, 13.7954)
  line L574 (-3.6275, 13.7954) -> (-18.6265, 13.7954)
  line L575 (-18.6265, 13.7954) -> (-18.6265, 13.4246)
  line L576 (-18.6265, 13.4246) -> (-18.6265, 0)
  line L577 (-18.6265, 0) -> (-18.6265, -1.2035)
  line L578 (-18.6265, -1.2035) -> (-18.1747, -1.2035)
  line L579 (-18.1747, -1.2035) -> (-4.1813, -1.2035)
  line L580 (-4.1813, -1.2035) -> (-3.6275, -1.2035)
  line L581 (-3.6275, -1.2035) -> (-3.6275, 0)
  line L582 (-3.6275, 0) -> (-3.6275, 13.4246)
  line L583 (-23.1726, 11.4254) -> (-32.7548, 11.4254)
  line L584 (-32.7548, 11.4254) -> (-37.167, 11.4254)
  line L585 (-37.167, 11.4254) -> (-37.167, 0)
  line L586 (-37.167, 0) -> (-37.167, -2.569)
  line L587 (-37.167, -2.569) -> (-32.7548, -2.569)
  line L588 (-32.7548, -2.569) -> (-23.1726, -2.569)
  line L589 (-23.1726, -2.569) -> (-23.1726, 0)
  line L590 (-23.1726, 0) -> (-23.1726, 11.4254)
  line L591 (-23.1726, 31.5173) -> (-32.7548, 31.5173)
  line L592 (-32.7548, 31.5173) -> (-37.167, 31.5173)
  line L593 (-37.167, 31.5173) -> (-37.167, 17.5229)
  line L594 (-37.167, 17.5229) -> (-32.7548, 17.5229)
  line L595 (-32.7548, 17.5229) -> (-23.1726, 17.5229)
  line L596 (-23.1726, 17.5229) -> (-23.1726, 19.4221)
  line L597 (-23.1726, 19.4221) -> (-23.1726, 31.5173)
  line L598 (-18.1747, -16.3774) -> (-18.1747, -20.5617)
  line L599 (-18.1747, -20.5617) -> (-4.1813, -20.5617)
  line L600 (-4.1813, -20.5617) -> (-4.1813, -16.3774)
  line L601 (-4.1813, -16.3774) -> (-4.1813, -6.5673)
  line L602 (-4.1813, -6.5673) -> (-18.1747, -6.5673)
  line L603 (-18.1747, -6.5673) -> (-18.1747, -16.3774)
  line L604 (-14.3112, -27.259) -> (-14.3112, -32.7548)
  line L605 (-14.3112, -32.7548) -> (-14.3112, -41.2533)
  line L606 (-14.3112, -41.2533) -> (-9.2832, -41.2533)
  line L607 (-9.2832, -41.2533) -> (-0.3179, -41.2533)
  line L608 (-0.3179, -41.2533) -> (-0.3179, -38.3862)
  line L609 (-0.3179, -38.3862) -> (-0.3179, -32.7548)
  line L610 (-0.3179, -32.7548) -> (-0.3179, -27.259)
  line L611 (-0.3179, -27.259) -> (-4.1813, -27.259)
  line L612 (-4.1813, -27.259) -> (-14.3112, -27.259)
  line L613 (-23.1726, -28.2052) -> (-32.7548, -29.8947)
  line L614 (-32.7548, -29.8947) -> (-35.2557, -30.3357)
  line L615 (-35.2557, -30.3357) -> (-34.8292, -32.7548)
  line L616 (-34.8292, -32.7548) -> (-32.8257, -44.1172)
  line L617 (-32.8257, -44.1172) -> (-32.7548, -44.1046)
  line L618 (-32.7548, -44.1046) -> (-19.0443, -41.6871)
  line L619 (-19.0443, -41.6871) -> (-19.1208, -41.2533)
  line L620 (-19.1208, -41.2533) -> (-20.6193, -32.7548)
  line L621 (-20.6193, -32.7548) -> (-21.4743, -27.9057)
  line L622 (-21.4743, -27.9057) -> (-23.1726, -28.2052)
  line L623 (-37.4649, -45.8135) -> (-37.9251, -45.0163)
  line L624 (-37.9251, -45.0163) -> (-44.462, -33.6934)
  line L625 (-44.462, -33.6934) -> (-49.1321, -36.3897)
  line L626 (-49.1321, -36.3897) -> (-56.5811, -40.6905)
  line L627 (-56.5811, -40.6905) -> (-56.4351, -40.9434)
  line L628 (-56.4351, -40.9434) -> (-51.7076, -49.1321)
  line L629 (-51.7076, -49.1321) -> (-49.584, -52.8106)
  line L630 (-49.584, -52.8106) -> (-49.1321, -52.5498)
  line L631 (-49.1321, -52.5498) -> (-43.2128, -49.1321)
  line L632 (-43.2128, -49.1321) -> (-37.4649, -45.8135)
  line L633 (51.0969, -40.9463) -> (52.5297, -32.8204)
  line L634 (52.5297, -32.8204) -> (53.6581, -26.4207)
  line L635 (53.6581, -26.4207) -> (39.1326, -23.8595)
  line L636 (39.1326, -23.8595) -> (38.6399, -26.654)
  line L637 (38.6399, -26.654) -> (37.9582, -30.5201)
  line L638 (37.9582, -30.5201) -> (37.5757, -32.6892)
  line L639 (37.5757, -32.6892) -> (36.5714, -38.3851)
  line L640 (36.5714, -38.3851) -> (49.0665, -40.5883)
  line L641 (49.0665, -40.5883) -> (51.0969, -40.9463)
  line L642 (55.4175, -16.443) -> (57.1297, -6.7317)
  line L643 (57.1297, -6.7317) -> (42.6042, -4.1705)
  line L644 (42.6042, -4.1705) -> (41.0793, -12.8194)
  line L645 (41.0793, -12.8194) -> (40.4635, -16.3118)
  line L646 (40.4635, -16.3118) -> (40.043, -18.697)
  line L647 (40.043, -18.697) -> (54.5684, -21.2582)
  line L648 (54.5684, -21.2582) -> (55.4175, -16.443)
  line L649 (58.3054, -0.0656) -> (60.6013, 12.9563)
  line L650 (60.6013, 12.9563) -> (46.0758, 15.5176)
  line L651 (46.0758, 15.5176) -> (43.5146, 0.991)
  line L652 (43.5146, 0.991) -> (51.245, -0.3721)
  line L653 (51.245, -0.3721) -> (58.0401, -1.5702)
  line L654 (58.0401, -1.5702) -> (58.3054, -0.0656)
  line L655 (-49.321, -36.0626) -> (-57.0972, -40.5523)
  line L656 (-57.0972, -40.5523) -> (-56.7623, -41.1323)
  line L657 (-56.7623, -41.1323) -> (-52.0348, -49.321)
  line L658 (-52.0348, -49.321) -> (-49.7222, -53.3267)
  line L659 (-49.7222, -53.3267) -> (-48.9432, -52.877)
  line L660 (-48.9432, -52.877) -> (-43.0239, -49.4593)
  line L661 (-43.0239, -49.4593) -> (-36.9488, -45.9518)
  line L662 (-36.9488, -45.9518) -> (-37.5979, -44.8274)
  line L663 (-37.5979, -44.8274) -> (-44.3237, -33.1773)
  line L664 (-44.3237, -33.1773) -> (-49.321, -36.0626)
  line L665 (33.8999, -26.6517) -> (34.7957, -16.4103)
  line L666 (34.7957, -16.4103) -> (35.1852, -11.9576)
  line L667 (35.1852, -11.9576) -> (34.5179, -11.8992)
  line L668 (34.5179, -11.8992) -> (32.7877, -11.7479)
  line L669 (32.7877, -11.7479) -> (20.4922, -10.6722)
  line L670 (20.4922, -10.6722) -> (19.9956, -16.3444)
  line L671 (19.9956, -16.3444) -> (19.2058, -25.3663)
  line L672 (19.2058, -25.3663) -> (32.7218, -26.5486)
  line L673 (32.7218, -26.5486) -> (33.8999, -26.6517)
  line L674 (35.3753, -6.4339) -> (35.9352, -0.0329)
  line L675 (35.9352, -0.0329) -> (36.6606, 8.2592)
  line L676 (36.6606, 8.2592) -> (32.7877, 8.5983)
  line L677 (32.7877, 8.5983) -> (22.3442, 9.5126)
  line L678 (22.3442, 9.5126) -> (21.9676, 9.5459)
  line L679 (21.9676, 9.5459) -> (21.4703, 3.8614)
  line L680 (21.4703, 3.8614) -> (21.1354, 0.0329)
  line L681 (21.1354, 0.0329) -> (20.6822, -5.1485)
  line L682 (20.6822, -5.1485) -> (32.7218, -6.2017)
  line L683 (32.7218, -6.2017) -> (35.3753, -6.4339)
  line L684 (37.1175, 13.4821) -> (37.368, 16.3444)
  line L685 (37.368, 16.3444) -> (38.4029, 28.1752)
  line L686 (38.4029, 28.1752) -> (32.7877, 28.6664)
  line L687 (32.7877, 28.6664) -> (23.7098, 29.4605)
  line L688 (23.7098, 29.4605) -> (22.4245, 14.7675)
  line L689 (22.4245, 14.7675) -> (32.7218, 13.8666)
  line L690 (32.7218, 13.8666) -> (37.1175, 13.4821)
  line L691 (15.1888, 18.2006) -> (0.4389, 18.2006)
  line L692 (0.4389, 18.2006) -> (0.4389, 3.4507)
  line L693 (0.4389, 3.4507) -> (15.1888, 3.4507)
  line L694 (15.1888, 3.4507) -> (15.1888, 18.2006)
  line L695 (0.4389, 32.7548) -> (0.4389, 31.084)
  line L696 (0.4389, 31.084) -> (0.4389, 23.4426)
  line L697 (0.4389, 23.4426) -> (15.1888, 23.4426)
  line L698 (15.1888, 23.4426) -> (15.1888, 29.8598)
  line L699 (15.1888, 29.8598) -> (15.1888, 32.7548)
  line L700 (15.1888, 32.7548) -> (15.1888, 38.1925)
  line L701 (15.1888, 38.1925) -> (0.4389, 38.1925)
  line L702 (0.4389, 38.1925) -> (0.4389, 32.7548)
  line L703 (15.1888, -1.7913) -> (0.4389, -1.7913)
  line L704 (0.4389, -1.7913) -> (0.4389, -16.5413)
  line L705 (0.4389, -16.5413) -> (15.1888, -16.5413)
  line L706 (15.1888, -16.5413) -> (15.1888, -1.7913)
  line L707 (-3.8035, -16.3774) -> (-3.8035, -6.1895)
  line L708 (-3.8035, -6.1895) -> (-18.5525, -6.1895)
  line L709 (-18.5525, -6.1895) -> (-18.5525, -16.3774)
  line L710 (-18.5525, -16.3774) -> (-18.5525, -20.9395)
  line L711 (-18.5525, -20.9395) -> (-3.8035, -20.9395)
  line L712 (-3.8035, -20.9395) -> (-3.8035, -16.3774)
  line L713 (-4.1813, -26.8812) -> (-14.689, -26.8812)
  line L714 (-14.689, -26.8812) -> (-14.689, -32.7548)
  line L715 (-14.689, -32.7548) -> (-14.689, -41.6311)
  line L716 (-14.689, -41.6311) -> (-9.2832, -41.6311)
  line L717 (-9.2832, -41.6311) -> (0.0599, -41.6311)
  line L718 (0.0599, -41.6311) -> (0.0599, -38.3862)
  line L719 (0.0599, -38.3862) -> (0.0599, -32.7548)
  line L720 (0.0599, -32.7548) -> (0.0599, -26.8812)
  line L721 (0.0599, -26.8812) -> (-4.1813, -26.8812)
  line L722 (-3.6275, -1.2036) -> (-3.6275, 0)
  line L723 (-3.6275, 0) -> (-3.6275, 13.4246)
  line L724 (-3.6275, 13.4246) -> (-3.6275, 13.7955)
  line L725 (-3.6275, 13.7955) -> (-18.6265, 13.7955)
  line L726 (-18.6265, 13.7955) -> (-18.6265, 13.4246)
  line L727 (-18.6265, 13.4246) -> (-18.6265, 0)
  line L728 (-18.6265, 0) -> (-18.6265, -1.2036)
  line L729 (-18.6265, -1.2036) -> (-18.1747, -1.2036)
  line L730 (-18.1747, -1.2036) -> (-4.1813, -1.2036)
  line L731 (-4.1813, -1.2036) -> (-3.6275, -1.2036)
  line L732 (-3.8035, 32.7548) -> (-3.8035, 33.7943)
  line L733 (-3.8035, 33.7943) -> (-8.1887, 33.7943)
  line L734 (-8.1887, 33.7943) -> (-16.3774, 33.7943)
  line L735 (-16.3774, 33.7943) -> (-18.5525, 33.7943)
  line L736 (-18.5525, 33.7943) -> (-18.5525, 32.7548)
  line L737 (-18.5525, 32.7548) -> (-18.5525, 19.0443)
  line L738 (-18.5525, 19.0443) -> (-3.8035, 19.0443)
  line L739 (-3.8035, 19.0443) -> (-3.8035, 32.7548)
  line L740 (-21.1679, -27.4681) -> (-23.2382, -27.8331)
  line L741 (-23.2382, -27.8331) -> (-32.8204, -29.5227)
  line L742 (-32.8204, -29.5227) -> (-35.6934, -30.0293)
  line L743 (-35.6934, -30.0293) -> (-35.2013, -32.8204)
  line L744 (-35.2013, -32.8204) -> (-33.1322, -44.5548)
  line L745 (-33.1322, -44.5548) -> (-32.6892, -44.4767)
  line L746 (-32.6892, -44.4767) -> (-18.6066, -41.9936)
  line L747 (-18.6066, -41.9936) -> (-18.7487, -41.1877)
  line L748 (-18.7487, -41.1877) -> (-20.2472, -32.6892)
  line L749 (-20.2472, -32.6892) -> (-21.1679, -27.4681)
  line L750 (-22.7948, -16.3774) -> (-22.7948, -8.1887)
  line L751 (-22.7948, -8.1887) -> (-32.7548, -8.1887)
  line L752 (-32.7548, -8.1887) -> (-37.5448, -8.1887)
  line L753 (-37.5448, -8.1887) -> (-37.5448, -16.3774)
  line L754 (-37.5448, -16.3774) -> (-37.5448, -22.9387)
  line L755 (-37.5448, -22.9387) -> (-32.7548, -22.9387)
  line L756 (-32.7548, -22.9387) -> (-22.7948, -22.9387)
  line L757 (-22.7948, -22.9387) -> (-22.7948, -16.3774)
  line L758 (-22.7948, 0) -> (-22.7948, 11.8032)
  line L759 (-22.7948, 11.8032) -> (-32.7548, 11.8032)
  line L760 (-32.7548, 11.8032) -> (-37.5448, 11.8032)
  line L761 (-37.5448, 11.8032) -> (-37.5448, 0)
  line L762 (-37.5448, 0) -> (-37.5448, -2.9468)
  line L763 (-37.5448, -2.9468) -> (-32.7548, -2.9468)
  line L764 (-32.7548, -2.9468) -> (-22.7948, -2.9468)
  line L765 (-22.7948, -2.9468) -> (-22.7948, 0)
  line L766 (-22.7948, 17.1451) -> (-22.7948, 19.4221)
  line L767 (-22.7948, 19.4221) -> (-22.7948, 31.8951)
  line L768 (-22.7948, 31.8951) -> (-32.7548, 31.8951)
  line L769 (-32.7548, 31.8951) -> (-37.5448, 31.8951)
  line L770 (-37.5448, 31.8951) -> (-37.5448, 17.1451)
  line L771 (-37.5448, 17.1451) -> (-32.7548, 17.1451)
  line L772 (-32.7548, 17.1451) -> (-22.7948, 17.1451)
  dimension "d2" = 0.1
  dimension "d3" = 0.1
  dimension "d4" = 0.1
  dimension "d15" = 0.1
  dimension "d16" = 0.1
  dimension "d17" = 0.1
  dimension "d18" = 0.1
  dimension "d19" = 0.1
  dimension "d20" = 0.1
  dimension "d21" = 0.1
  dimension "d22" = 0.1
  dimension "d23" = 0.1
  dimension "d24" = 0
  dimension "d25" = 0.1
  dimension "d26" = 0.1
  dimension "d27" = 0.1
  dimension "d28" = 0.1
  dimension "d29" = 0.1
scale "Scale1" [no effect]
extrude "Extrude6" add sketch "Sketch1" along normal blind 1.5 contours L0 L1 L2 L3 L4 L5 L6 L7 L8 L9 L10 L11 L12 L13 L14 L15 L16 L17 L18 L19 L20 L21 L22 L23 L24 L25 L26 L27 L28 L29 L30 L31 L32 L33 L34 L35 L36 L37 L38 L39 L40 L41 L42 L43 L44 L45 L46 L47 L48 L49 L50 L51 L52 L53 L54 L55 L56 L57 L58 L59 L60 L61 L62 L63 L64 L65 L66 L67 L68 L69 L70 L71 L72 L73 L74 L75 L76 L77 L78 L79 L80 L81 L82 L84 L85 L86 L87 L88 L89 L90 L91 L92 L93 L94 L95 L96 L97 L98 L99 L100 L101 L102 L103 L104 L105 L106 L107 L108 L109 L111 L112 L113 L114 L115 L116 L117 L118 L119 L120 L121 L122 L123 L124 L125 L126 L127 L128 L129 L130 L131 L132 L133 L134 L135 L136 L137 L138 L139 L140 L141 L142 L143 L144 L145 L146 L147 L148 L149 L150 L151 L152 L153 L154 L155 L156 L157 L158 L159 L160 L161 L162 L163 L164 L165 L166 L167 L168 L169 L170 L171 L172 L173 L174 L175 L176 L177 L178 L179 L180 L181 L182 L183 L184 L185 L186 L187 L188 L189 L190 L191 L192 L193 L194 L195 L196 L197 L198 L199 L200 L201 L202 L203 L204 L205 L206 L207 L208 L209 L210 L211 L212 L213 L214 L215 L216 L217 L218 L219 L220 L221 L222 L223 L224 L225 L226 L227 L228 L229 L230 L231 L232 L233 L234 L235 L236 L237 L238 L239 L240 L241 L242 L243 L244 L245 L246 L247 L248 L249 L250 L251 L252 L253 L254 L255 L256 L257 L258 L259 L260 L261 L262 L263 L264 L265 L266 L267 L268 L269 L270 L271 L272 L273 L274 L275 L276 L277 L278 L279 L280 L281 L282 L283 L284 L285 L286 L287 L288 L289 L290 L291 L292 L293 L294 L295 L296 L297 L298 L299 L300 L301 L302 L303 L304 L305 L306 L307 L308 L309 L310 L311 L312 L313 L314 L315 L316 L317 L318 L319 L320 L321 L322 L323 L324 L325 L326 L327 L328 L329 L330 L331 L332 L333 L334 L335 L336 L337 L338 L339 L340 L341 L342 L343 L344 L345 L346 L347 L348 L349 L350 L351 L352 L353 L354 L355 L356 L357 L358 L359 L360 L361 L362 L363 L364 L365 L366 L367 L368 L369 L370 L371 L372 L373 L374 L375 L376 L377 L378 L379 L380 L381 L382 L383 L384 L385 L386 L387 L388 L389 L390 L391 L392 L393 L394 L395 L396 L397 L398 L399 L400 L401 L402 L403 L404 L405 L406 L407 L408 L409 L410 L411 L412 L413 L414 L415 L416 L417 L418 L419 L420 L421 L422 L423 L424 L425 L426 L427 L428 L429 L430 L431 L432 L433 L434 L435 L436 L437 L438 L439 L440 L441 L442 L443 L444 L445 L446 L447 L448 L449 L450 L451 L452 L453 L454 L455 L456 L457 L458 L459 L460 L461 L462 L463 L464 L465 L466 L467 L468 L469 L470 L471 L472 L473 L474 L475 L476 L477 L478 L479 L480 L481 L482 L483 L484 L485 L486 L487 L488 L489 L490 L491 L492
